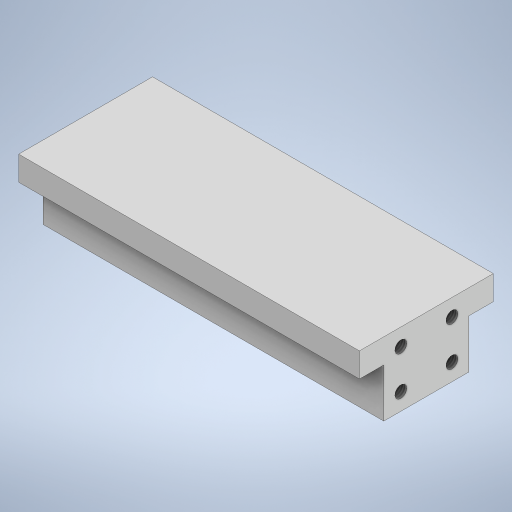
# Autodesk Inventor part: Fuhrung
Saved by Autodesk Inventor 2024 (Build 280153000, 153)
## iProperties
Created: 2023-05-10
Part Number: Fuhrung
Material: Generic
Document SubType Name: Modeling
Designer: Raj
Density: 1 g/cm^3
Appearance: Default
Author: Raj
Autodesk Inventor part; units mm, degrees
ref_plane "YZ Plane" through (0, 0, 0) normal (1, 0, 0) x (0, 1, 0)
ref_plane "XZ Plane" through (0, 0, 0) normal (0, 1, 0) x (-1, 0, 0)
ref_plane "XY Plane" through (0, 0, 0) normal (0, 0, 1) x (1, 0, 0)
sketch "Sketch1" plane through (0, 0, 0) normal (0, 0, 1) x (1, 0, 0)
  line L0 (-70, 17.5) -> (70, 17.5)
  line L1 (70, 17.5) -> (70, -17.5)
  line L2 (70, -17.5) -> (-70, -17.5)
  line L3 (-70, -17.5) -> (-70, 17.5)
  line L4 (-70, 17.5) -> (70, -17.5) construction
  line L5 (70, 17.5) -> (-70, -17.5) construction
  point P0 (0, 0)
  dimension "d0" = 140
  dimension "d1" = 35
  constraints: 12 end point, 2 midpoint, 2 parallel, 1 horizontal, 1 perpendicular
  measures "d0" distance of L1.end L2.end
  measures "d1" distance of L0.end L1.end
extrude "Extrusion1" add sketch "Sketch1" along normal blind 20
sketch "Sketch2" plane through (0, 0, 20) normal (0, 0, 1) x (1, 0, 0)
  line L0 (70, -27.5) -> (-70, -27.5)
  line L1 (-70, -27.5) -> (-70, 27.5)
  line L2 (-70, 27.5) -> (70, 27.5)
  line L3 (70, 27.5) -> (70, -27.5)
  line L4 (70, -27.5) -> (-70, 27.5) construction
  line L5 (-70, -27.5) -> (70, 27.5) construction
  point P0 (0, 0)
  dimension "d4" = 140
  dimension "d5" = 55
  constraints: 12 end point, 2 midpoint, 2 parallel, 1 horizontal, 1 perpendicular
  measures "d4" distance of L1.end L2.end
  measures "d5" distance of L0.end L1.end
extrude "Extrusion2" add sketch "Sketch2" along normal blind 10
sketch "Sketch4" plane through (70, -17.5, 0) normal (1, 0, 0) x (0, 0, -1)
  line L0 (0, 0) -> (0, 35) projected
  point P0 (0, 17.5)
  point P1 (-7, 28)
  point P2 (0, 17.5)
  dimension "d24" = 10.5
  dimension "d25" = 7
  constraints: 1 midpoint
  measures "d24" vertical distance of point (-7, 28) point (0, 17.5)
  measures "d25" distance from line of point (-7, 28) L0
hole "Hole2" at (70, 10.5, 7) direction (-1, 0, 0) diameter 4.917 depth 20 tip angle 118 thread size "M6x1" class "6H" standard "ISO Metric profile"
pattern_linear "Rectangular Pattern2" count 2 spacing 16 along (0, 0, 1) count 2 spacing 21 along (0, -1, 0) of "Hole2"
sketch "Sketch5" plane through (-70, -17.5, 0) normal (-1, 0, 0) x (0, 0, 1)
  line L0 (0, 35) -> (0, 0) projected
  line L1 (0, 17.5) -> (33.2341, 17.5) construction
  point P0 (0, 17.5)
  point P1 (8, 17.5)
  point P2 (23, 28)
  point P3 (23, 7)
  dimension "d39" = 8
  dimension "d40" = 15
  dimension "d41" = 15
  dimension "d42" = 10.5
  dimension "d43" = 10.5
  constraints: 2 end point, 1 horizontal, 1 midpoint
  measures "d39" distance of L1.start point (8, 17.5)
  measures "d40" horizontal distance of point (8, 17.5) point (23, 28)
  measures "d41" horizontal distance of point (8, 17.5) point (23, 7)
  measures "d42" distance from line of point (23, 28) L1
  measures "d43" distance from line of L1 point (23, 7)
hole "Hole3" at (-70, 0, 8) at (-70, 10.5, 23) at (-70, -10.5, 23) direction (1, 0, 0) diameter 6.647 depth 20 tip angle 118 thread size "M8x1.25" class "6H" standard "ISO Metric profile"
sketch "Sketch6" plane through (0, 0, 0) normal (0, 0, -1) x (-1, 0, 0)
  line L0 (-70, -17.5) -> (-70, 17.5) projected
  point P0 (0, 0)
  point P1 (-45, -12.5)
  dimension "d51" = 25
  dimension "d52" = 12.5
  measures "d51" distance from line of point (-45, -12.5) L0
  measures "d52" vertical distance of point (-45, -12.5) point (0, 0)
hole "Hole4" at (45, -12.5, 0) direction (0, 0, 1) diameter 4.917 depth 15 tip angle 118 thread size "M6x1" class "6H" standard "ISO Metric profile"
pattern_linear "Rectangular Pattern3" count 3 spacing 45 along (-1, 0, 0) count 2 spacing 25 along (0, 1, 0) of "Hole4"
body "Solid1"
